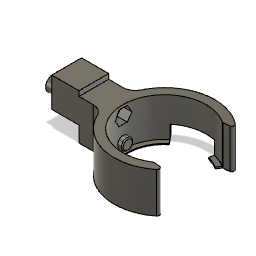
_3rd Tube Connector.98e6ea30-230d-4ec6-be3d-76e0818ba304 (Autodesk Fusion 360 design; units mm, degrees)
Autodesk Fusion 360 part; units mm, degrees
note: some values were not read from the file. Set by a fixed rule: which sketch regions a step uses.
sketch "Sketch1" plane through (0, 0, 0) normal (0, 1, 0) x (1, 0, 0)
  line L0 (-39.5, 0) -> (-39.5, 6)
  line L1 (-39.5, 6) -> (-22.7835, 6)
  line L2 (-50, 0) -> (42, 0) construction
  line L3 (0, 0) -> (18.7964, 26.8441) construction
  arc A0 (9.1081, 14.1168) -> (-16.8, 0) centre (0, 0) ccw
  arc A1 (12.6271, 15.8949) -> (-18.2809, 8.8261) centre (0, 0) ccw
  arc A2 (-22.7835, 6) -> (-18.2809, 8.8261) centre (-22.7835, 11) ccw
  line L4 (-28.5277, 8) -> (-28.5277, 0)
  line L5 (-39.5, -6) -> (-22.7835, -6)
  arc A3 (-18.2809, -8.8261) -> (12.6271, -15.8949) centre (0, 0) ccw
  arc A4 (-18.2809, -8.8261) -> (-22.7835, -6) centre (-22.7835, -11) ccw
  line L6 (-28.5277, -8) -> (-28.5277, 0)
  arc A5 (-16.8, 0) -> (9.1081, -14.1168) centre (0, 0) ccw
  line L7 (-39.5, 0) -> (-39.5, -6)
  arc A6 (9.5679, 13.9604) -> (12.2171, 14.1346) centre (10.3084, 22.9299) ccw
  line L8 (0, 28) -> (0, 20.2823) construction
  line L9 (0, 20.3) -> (0, -24) construction
  arc A7 (12.2171, 14.1346) -> (12.6271, 15.8949) centre (12.005, 15.1119) ccw
  arc A8 (9.1081, 14.1168) -> (9.5679, 13.9604) centre (9.6502, 14.957) ccw
  arc A9 (12.6271, -15.8949) -> (12.2171, -14.1346) centre (12.005, -15.1119) ccw
  arc A10 (12.2171, -14.1346) -> (9.5679, -13.9604) centre (10.3084, -22.9299) ccw
  arc A11 (9.5679, -13.9604) -> (9.1081, -14.1168) centre (9.6502, -14.957) ccw
  point P0 (-50, 0)
  dimension "d1" = 33.6
  dimension "d4" = 6
  dimension "d5" = 39.5
  dimension "d6" = 3.5
  dimension "d7" = 5
  dimension "d11" = 55
  dimension "d30" = 1
  dimension "d31" = 9
  dimension "d32" = 1
  constraint coincident L3.start A0.centre
  constraint vertical L0
  constraint perpendicular L0 L1
  constraint horizontal L2
  constraint vertical L8
  constraint coincident L0.start L2
  constraint coincident L2 A0.end
  constraint tangent A1 A2
  constraint tangent L1 A2
  constraint coincident L2 L4.end
  constraint perpendicular L2 L4
  constraint symmetric L3.start L2 A0.centre
  constraint symmetric L0.start L2 L7.start
  constraint symmetric L0.end L2 L5.start
  constraint symmetric P0 L2 L2.start
  constraint symmetric L2 L3.start A0.centre
  constraint symmetric L2 A0.end A5.start
  constraint symmetric L2 A0 A5
  constraint symmetric L2 A1 A3
  constraint symmetric L2 L1.end L5.end
  constraint symmetric L2 A1.end A3.start
  constraint symmetric L2 A2 A4
  constraint symmetric L2 L4.start L6.start
  constraint symmetric L2 L4.end L6.end
  constraint coincident A1 L9.start
  constraint collinear L8 L9
  constraint tangent A1 A7
  constraint tangent A6 A7
  constraint tangent A6 A8
  constraint tangent A0 A8
  constraint equal A7 A8
  constraint symmetric L2 A6 A10
  constraint symmetric L2 A1.start A3.end
  constraint symmetric L2 A6.end A9.end
  constraint symmetric L2 A7 A9
  constraint tangent A10 A11
  constraint tangent A5 A11
  measures "d1" diameter of A0
  measures "d4" distance of L0.start L0.end
  measures "d5" distance of L3.start L0
  measures "d6" distance of A0 A1
  measures "d7" radius of A2
  measures "d11" angle of L2 L3
  measures "d30" radius of A7
  measures "d31" radius of A6
  measures "d32" radius of A11
extrude "Extrude1" add sketch "Sketch1" along normal blind 4 and the other way blind 12.25 contours L1 A0 A1 A2 L4 L5 A3 A4 L6 A5 A6 A7 A8 A9 A10 A11
extrude "Extrude2" add sketch "Sketch1" along normal mid plane 12 contours L0 L1 L4 L5 L6 L7
ref_plane "WorkPlane1" through (-16.8, 0, 0) normal (1, 0, 0) x (0, 1, 0)
sketch "Sketch2" plane through (-16.8, 0, 0) normal (1, 0, 0) x (0, 0, -1)
  line L0 (-1.6743, 2.9) -> (-3.3486, 0)
  line L1 (-3.3486, 0) -> (-1.6743, -2.9)
  line L2 (-1.6743, -2.9) -> (1.6743, -2.9)
  line L3 (1.6743, -2.9) -> (3.3486, 0)
  line L4 (3.3486, 0) -> (1.6743, 2.9)
  line L5 (1.6743, 2.9) -> (-1.6743, 2.9)
  circle A0 centre (0, 0) radius 1.65
  line L6 (2.175, 2.175) -> (-2.175, -2.175) construction
  line L7 (-2.175, 2.175) -> (2.175, -2.175) construction
  dimension "d16" = 2.9
  dimension "d25" = 3.3
  dimension "d45" = 4.35
  dimension "d46" = 4.35
  constraint coincident A0.centre origin
  constraint coincident L6 A0.centre
  constraint coincident L7 A0.centre
  measures "d16" distance of A0.centre L5
  measures "d25" diameter of A0
  measures "d45" distance of L6.end L7.end
  measures "d46" distance of L7.start L6.end
extrude "Extrude3" cut sketch "Sketch2" along normal blind 1 and the other way blind 4 contours L0 L1 L2 L3 L4 L5 | A0
sketch "Sketch3" plane through (-39.5, 0, 0) normal (-1, 0, 0) x (0, 0, 1)
  line L0 (6, -6) -> (6, 6)
  line L1 (6, 6) -> (-6, 6)
  line L2 (-6, 6) -> (-6, -6)
  line L3 (-6, -6) -> (6, -6)
  line L4 (2.5, 3) -> (-2.5, 3)
  arc A0 (-2.5, 3) -> (-2.5, -3) centre (-2.5, 0) ccw
  line L5 (-2.5, -3) -> (2.5, -3)
  arc A1 (2.5, -3) -> (2.5, 3) centre (2.5, 0) ccw
  line L6 (2.5, 0) -> (-2.5, 0) construction
  dimension "d64" = 5
  dimension "d65" = 6
  constraint tangent L4 A0
  constraint tangent A0 L5
  constraint parallel L4 L5
  constraint tangent L5 A1
  constraint tangent L4 A1
  constraint perpendicular L0 L6
  constraint midpoint L6 origin
  measures "d64" distance of A1.centre A0.centre
  measures "d65" distance of L4 L5
extrude "Extrude4" add sketch "Sketch3" along normal blind 3 contours L4 A0 L5 A1
extrude "Extrude5" cut sketch "Sketch2" against normal blind 45 contours A0
sketch "Sketch5" plane through (0, -12.25, 0) normal (0, -1, 0) x (1, 0, 0)
  line L0 (-28.5277, 6) -> (-28.5277, -6)
  arc A0 (12.6271, -15.8949) -> (12.2171, -14.1346) centre (12.005, -15.1119) ccw
  arc A1 (12.2171, -14.1346) -> (9.5679, -13.9604) centre (10.3084, -22.9299) ccw
  arc A2 (9.5679, 13.9604) -> (12.2171, 14.1346) centre (10.3084, 22.9299) ccw
  arc A3 (12.2171, 14.1346) -> (12.6271, 15.8949) centre (12.005, 15.1119) ccw
  arc A4 (12.6271, 15.8949) -> (-18.2809, 8.8261) centre (0, 0) ccw
  arc A5 (-22.7835, 6) -> (-18.2809, 8.8261) centre (-22.7835, 11) ccw
  line L1 (-22.7835, 6) -> (-28.5277, 6)
  line L2 (-28.5277, -6) -> (-22.7835, -6)
  arc A6 (-18.2809, -8.8261) -> (-22.7835, -6) centre (-22.7835, -11) ccw
  arc A7 (-18.2809, -8.8261) -> (12.6271, -15.8949) centre (0, 0) ccw
  arc A8 (9.5679, -13.9604) -> (9.1081, -14.1168) centre (9.6502, -14.957) ccw
  arc A9 (9.1081, 14.1168) -> (9.1081, -14.1168) centre (0, 0) ccw
  arc A10 (9.1081, 14.1168) -> (9.5679, 13.9604) centre (9.6502, 14.957) ccw
  arc A11 (9.1081, 14.1168) -> (9.1081, -14.1168) centre (0, 0) ccw
  arc A12 (9.6502, 14.957) -> (9.6502, -14.957) centre (0, 0) ccw
  arc A13 (8.0238, 12.4362) -> (8.0238, -12.4362) centre (0, 0) ccw
  line L3 (8.0238, 12.4362) -> (9.1081, 14.1168)
  line L4 (8.0238, -12.4362) -> (9.1081, -14.1168)
  dimension "d37" = 1
  dimension "d38" = -2
  constraint coincident A9.start A10.start
  constraint coincident A8.end A9.end
extrude "Extrude6" add sketch "Sketch5" against normal blind 0.65 contours A9 A11 A13 L3 L4
sketch "Sketch6" plane through (0, -12.25, 0) normal (0, -1, 0) x (1, 0, 0)
  arc A0 (12.6271, 15.8949) -> (-18.2809, 8.8261) centre (0, 0) ccw
  arc A1 (-22.7835, 6) -> (-18.2809, 8.8261) centre (-22.7835, 11) ccw
  line L0 (-22.7835, 6) -> (-28.5277, 6)
  line L1 (-28.5277, 6) -> (-28.5277, -6)
  line L2 (-28.5277, -6) -> (-22.7835, -6)
  arc A2 (-18.2809, -8.8261) -> (-22.7835, -6) centre (-22.7835, -11) ccw
  arc A3 (-18.2809, -8.8261) -> (12.6271, -15.8949) centre (0, 0) ccw
  arc A4 (12.6271, -15.8949) -> (12.2171, -14.1346) centre (12.005, -15.1119) ccw
  arc A5 (12.2171, -14.1346) -> (9.5679, -13.9604) centre (10.3084, -22.9299) ccw
  arc A6 (9.5679, -13.9604) -> (9.1081, -14.1168) centre (9.6502, -14.957) ccw
  line L3 (9.1081, -14.1168) -> (8.0238, -12.4362)
  arc A7 (8.0238, 12.4362) -> (8.0238, -12.4362) centre (0, 0) ccw
  line L4 (8.0238, 12.4362) -> (9.1081, 14.1168)
  arc A8 (9.1081, 14.1168) -> (9.5679, 13.9604) centre (9.6502, 14.957) ccw
  arc A9 (9.5679, 13.9604) -> (12.2171, 14.1346) centre (10.3084, 22.9299) ccw
  arc A10 (12.2171, 14.1346) -> (12.6271, 15.8949) centre (12.005, 15.1119) ccw
  arc A11 (8.0238, 12.4362) -> (8.0238, -12.4362) centre (0, 0) ccw
  arc A12 (-18.2809, -8.8261) -> (12.6271, -15.8949) centre (0, 0) ccw
  line L5 (4.5, -19.7949) -> (0, 0)
  line L6 (0, 0) -> (-13, -15.5913)
  line L7 (0, 0) -> (0, -26.4362)
  point P0 (0, -20.3)
  dimension "d41" = 4.5
  dimension "d42" = 13
  constraint coincident A3 L5.start
  constraint coincident A0.centre A3.centre
  constraint coincident A3 L6.end
  constraint vertical L7
  constraint coincident L7 P0
  constraint coincident A12 P0
  measures "d41" horizontal distance of L5.start P0
  measures "d42" horizontal distance of L6.end P0
extrude "Extrude7" cut sketch "Sketch6" against normal blind 6 contours A3 A7 A11 A12 L6 L7 | A3 A7 A11 A12 L5 L7
sketch "Sketch7" plane through (0, 0, 0) normal (0, 0, 1) x (1, 0, 0)
sketch "Sketch8" plane through (-16.8, 0, 0) normal (1, 0, 0) x (0, 0, -1)
  line L0 (0, 10) -> (0, -14) construction
  line L1 (23, 0) -> (-23, 0)
  line L2 (1.175, -5.45) -> (-1.175, -5.45)
  line L3 (-2.175, -6.45) -> (-2.175, -8.8)
  line L4 (-1.175, -9.8) -> (1.175, -9.8)
  line L5 (2.175, -8.8) -> (2.175, -6.45)
  line L6 (2.175, -5.45) -> (-2.175, -9.8) construction
  line L7 (-2.175, -5.45) -> (2.175, -9.8) construction
  line L8 (-14.8, -11.6) -> (11.3671, -11.6)
  arc A0 (-1.175, -5.45) -> (-2.175, -6.45) centre (-1.175, -6.45) ccw
  arc A1 (2.175, -6.45) -> (1.175, -5.45) centre (1.175, -6.45) ccw
  arc A2 (1.175, -9.8) -> (2.175, -8.8) centre (1.175, -8.8) ccw
  arc A3 (-2.175, -8.8) -> (-1.175, -9.8) centre (-1.175, -8.8) ccw
  circle A4 centre (0, -8.9881) radius 2.25
  point P0 (0, -7.625)
  dimension "d54" = 4.35
  dimension "d55" = 4.35
  dimension "d56" = 1.8
  dimension "d57" = 1
  dimension "d58" = 1
  dimension "d69" = 4.5
  constraint vertical L0
  constraint horizontal L1
  constraint horizontal L2
  constraint perpendicular L2 L3
  constraint parallel L2 L4
  constraint parallel L3 L5
  constraint coincident L6 P0
  constraint coincident L7 P0
  constraint coincident L0 P0
  constraint coincident L7.start L2
  constraint coincident L7.start L3
  constraint tangent L2 A0
  constraint tangent L3 A0
  constraint coincident L6.start L5
  constraint coincident L6.start L2
  constraint tangent L5 A1
  constraint tangent L2 A1
  constraint equal A0 A1
  constraint coincident L7.end L5
  constraint coincident L7.end L4
  constraint tangent L5 A2
  constraint tangent L4 A2
  constraint coincident L6.end L3
  constraint coincident L6.end L4
  constraint tangent L3 A3
  constraint tangent L4 A3
  constraint equal A2 A3
  constraint coincident L0 A4.centre
  measures "d54" distance of L6.end L7.end
  measures "d55" distance of L7.start L6.end
  measures "d56" distance of L4 L8
  measures "d57" radius of A0
  measures "d58" radius of A2
  measures "d69" diameter of A4
extrude "Extrude9" add sketch "Sketch8" along normal blind 2 contours L3 L4 L5 A2 A3 A4 | L3 L4 L5 A2 A3 A4
fillet "Fillet5" radius 0.4 1 faces at (-14.8, -9.4982, -0.6896)
chamfer "Chamfer1" distance 0.5 angle 35 8 edges at (-25.6556, -12.25, -6) (-20.1255, -12.25, -6.7651) (-16.002, -12.25, -12.491) (-11.9238, -12.25, 8.7671) (8.7827, -12.25, -18.3017) (12.979, -12.25, -14.8851) (10.899, -12.25, -13.9493) (9.3284, -12.25, -14.0103) measured on face at (-19.6564, -12.25, -0.0644) measured on face at (-19.6564, -12.25, -0.0644) measured on face at (-19.6564, -12.25, -0.0644) measured on face at (-11.4701, -12.0333, -9.3529) measured on face at (5.6098, -12.25, -17.5511) measured on face at (5.6098, -12.25, -17.5511) measured on face at (5.6098, -12.25, -17.5511) measured on face at (5.6098, -12.25, -17.5511)
equation "d5 = 50 mm - 10.5 mm"
equation "d35 = 4 mm + 9 mm - 0.75 mm"
